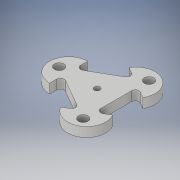
# Autodesk Inventor part: 80_20_Connector
Saved by Autodesk Inventor 2019 (Build 230136000, 136)
## iProperties
Created: 2019-07-24
Part Number: 80_20_Connector
Material: Generic
Document SubType Name: Modeling
Designer: Jorian Brusind
Density: 1 g/cm^3
Appearance: Default
Author: Jorian Brusind
Autodesk Inventor part; units mm, degrees
ref_plane "YZ Plane" through (0, 0, 0) normal (1, 0, 0) x (0, 1, 0)
ref_plane "XZ Plane" through (0, 0, 0) normal (0, 1, 0) x (-1, 0, 0)
ref_plane "XY Plane" through (0, 0, 0) normal (0, 0, 1) x (1, 0, 0)
sketch "Sketch1" plane through (0, 0, 0) normal (0, 1, 0) x (-1, 0, 0)
  circle A0 centre (0, 0) radius 20
  line L0 (0, 0) -> (20, 0)
  line L1 (20, 0) -> (-10, 17.3205)
  line L2 (20, 0) -> (54.641, 0) construction
  line L3 (-10, 17.3205) -> (-10, -17.3205)
  line L4 (20, 0) -> (-10, -17.3205)
  line L5 (0, 0) -> (12, 0)
  dimension "d0" = 40
  dimension "d1" = 150
  dimension "d2" = 12
  constraints: 12 end point, 3 point on circle, 2 horizontal, 1 centre point, 1 coincident, 1 equal length, 1 point on line, 1 vertical
  measures "d0" diameter of A0
  measures "d1" angle of L2 L1
  measures "d2" distance of L0.start L5.end
extrude "Extrusion1" add sketch "Sketch1" along normal blind 5 contours L4 L3 L1
sketch "Sketch2" plane through (0, 5, 0) normal (0, 1, 0) x (1, 0, 0)
  line L0 (0, 0) -> (-15, 0)
  arc A0 (-15, 10) -> (-15, -10) centre (-15, 0) ccw
  line L1 (-15, 0) -> (-15, -10)
  line L2 (-15, 0) -> (-15, 10)
  dimension "d5" = 15
  dimension "d7" = 10
  constraints: 6 end point, 2 point on circle, 1 centre point, 1 coincident, 1 collinear, 1 horizontal, 1 vertical
  measures "d5" distance of L0.start L0.end
  measures "d7" radius of A0
extrude "Extrusion2" add sketch "Sketch2" against normal blind 5
sketch "Sketch3" plane through (0, 5, 0) normal (0, 1, 0) x (1, 0, 0)
  circle A0 centre (0, 0) radius 1.5
  dimension "d10" = 3
  constraints: 1 centre point, 1 coincident
  measures "d10" diameter of A0
extrude "Extrusion3" cut sketch "Sketch3" against normal blind 5
pattern_circular "Circular Pattern1" count 3 over 360 about axis through (0, 5, 0) along (0, -1, 0) of "Extrusion2"
sketch "Sketch4" plane through (0, 5, 0) normal (0, 1, 0) x (1, 0, 0)
  circle A0 centre (0, 0) radius 1.5 projected
  line L0 (0, 0) -> (-20, 0)
  circle A1 centre (-20, 0) radius 2.5
  dimension "d16" = 20
  dimension "d17" = 5
  constraints: 2 end point, 1 centre point, 1 coincident, 1 horizontal
  measures "d16" distance of L0.start L0.end
  measures "d17" diameter of A1
extrude "Extrusion4" cut sketch "Sketch4" against normal blind 5 contours A1
pattern_circular "Circular Pattern2" count 3 over 360 about axis through (0, 5, 0) along (0, -1, 0) of "Extrusion4"
fillet "Fillet1" radius 2 6 edges at (5, 2.5, -14.4338) (10, 2.5, -11.547) (-15, 2.5, -2.8868) (-15, 2.5, 2.8868) (5, 2.5, 14.4338) (10, 2.5, 11.547)
body "Solid1"
